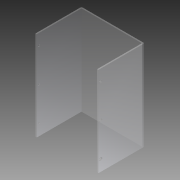
# Autodesk Inventor part: 13_0204_059
Saved by Autodesk Inventor 2012 SP1 (Build 160190100, 190)
## iProperties
Created: 2013-04-16
Part Number: 13_0204_059
Material: Default
Document SubType Name: Modeling
Designer: vogel
Density: 1 g/cm^3
Author: vogel
Autodesk Inventor part; units mm, degrees
ref_plane "YZ Plane" through (0, 0, 0) normal (1, 0, 0) x (0, 1, 0)
ref_plane "XZ Plane" through (0, 0, 0) normal (0, 1, 0) x (-1, 0, 0)
ref_plane "XY Plane" through (0, 0, 0) normal (0, 0, 1) x (1, 0, 0)
sketch "Skizze1" plane through (0, 0, 0) normal (0, 0, 1) x (1, 0, 0)
  line L0 (-99.5698, 0) -> (99.5698, 0) projected
  line L1 (0, -20.7243) -> (0, 124.3456) projected
  line L2 (67.5, 0) -> (67.5, 100)
  line L3 (67.5, 100) -> (-67.5, 100)
  line L4 (-67.5, 100) -> (-67.5, 0)
  line L5 (67.5, 0) -> (70.5, 0)
  line L6 (70.5, 0) -> (70.5, 100)
  line L7 (67.5, 103) -> (-67.5, 103)
  line L8 (-70.5, 100) -> (-70.5, 0)
  line L9 (-70.5, 0) -> (-67.5, 0)
  arc A0 (-67.5, 103) -> (-70.5, 100) centre (-67.5, 100) ccw
  arc A1 (70.5, 100) -> (67.5, 103) centre (67.5, 100) ccw
  point P0 (0, 0)
  dimension "d0" = 135
  dimension "d1" = 3
  dimension "d2" = 100
  dimension "d3" = 3
  dimension "d4" = 3
  constraints: 16 end point, 4 point on circle, 4 tangent, 3 parallel, 2 centre point, 2 collinear, 2 point on line, 1 equal radius, 1 horizontal, 1 perpendicular, 2 other
  measures "d0" distance between parallel lines of L2 L4
  measures "d1" distance of L8.end L4.end
  measures "d2" distance between parallel lines of L0 L3
  measures "d3" distance between parallel lines of L7 L3
  measures "d4" radius of A0
extrude "Extrusion1" add sketch "Skizze1" along normal blind 200 contours L8 A0 L7 L1 L3 L4 L0 | L2 L3 L1 L7 A1 L6 L0
sketch "Skizze2" plane through (70.5, 0, 0) normal (1, 0, 0) x (0, 0, -1)
  line L0 (-200, 100) -> (-200, 0) projected
  line L1 (0, 0) -> (-200, 0) projected
  line L2 (0, 0) -> (0, 100) projected
  line L3 (0, 100) -> (-200, 100) projected
  line L4 (-200, 5) -> (0, 5)
  line L5 (-100, 100) -> (-100, 0)
  point P0 (-175, 5)
  point P1 (-25, 5)
  point P2 (-100, 5)
  dimension "d7" = 5
  dimension "d8" = 25
  dimension "d9" = 25
  constraints: 5 point on line, 4 end point, 3 midpoint, 1 perpendicular
  measures "d7" distance between parallel lines of L4 L1
  measures "d8" distance from line of L0 point (-175, 5)
  measures "d9" distance of L4.end point (-25, 5)
hole "Bohrung1" at (70.5, 5, 175) at (70.5, 5, 25) at (70.5, 5, 100) direction (-1, 0, 0) diameter 3.4 end through all countersink diameter 6.9 countersink angle 90
sketch "Skizze3" plane through (-70.5, 0, 0) normal (-1, 0, 0) x (0, 0, 1)
  circle A0 centre (100, 5) radius 1.7 projected
  circle A1 centre (25, 5) radius 1.7 projected
  circle A2 centre (175, 5) radius 1.7 projected
  point P0 (25, 5)
  point P1 (100, 5)
  point P2 (175, 5)
  constraints: 3 coincident
hole "Bohrung2" at (-70.5, 5, 25) at (-70.5, 5, 100) at (-70.5, 5, 175) direction (1, 0, 0) diameter 3.4 end through all countersink diameter 6.9 countersink angle 90
